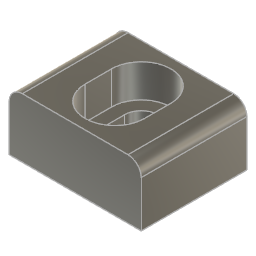
ZAxis Cap (Autodesk Fusion 360 design; units mm, degrees)
Autodesk Fusion 360 part; units mm, degrees
sketch "Sketch1" plane through (0, 0, 0) normal (0, 0, 1) x (1, 0, 0)
  line L0 (0, 0) -> (20, 0)
  line L1 (20, 0) -> (20, -16)
  line L2 (20, -16) -> (0, -16)
  line L3 (0, -16) -> (0, 0)
  line L4 (20, -8) -> (0, -8) construction
  line L5 (10, 0) -> (10, -16) construction
  line L6 (7.5, -6) -> (7.5, -10)
  arc A0 (7.5, -10) -> (12.5, -10) centre (10, -10) ccw
  line L7 (12.5, -10) -> (12.5, -6)
  arc A1 (12.5, -6) -> (7.5, -6) centre (10, -6) ccw
  line L8 (10, -6) -> (10, -10) construction
  line L9 (5.5, -6) -> (5.5, -10)
  arc A2 (5.5, -10) -> (14.5, -10) centre (10, -10) ccw
  line L10 (14.5, -10) -> (14.5, -6)
  arc A3 (14.5, -6) -> (5.5, -6) centre (10, -6) ccw
  line L11 (10, -6) -> (10, -10) construction
  dimension "d1" = 20
  dimension "d2" = 16
  dimension "d11" = 5
  dimension "d12" = 2
  dimension "d13" = 2
  dimension "d14" = 9
  constraint horizontal L0
  constraint vertical L1
  constraint horizontal L2
  constraint vertical L3
  constraint coincident L0.start L3.end
  constraint midpoint L1 L4.start
  constraint midpoint L3 L4.end
  constraint midpoint L0 L5.start
  constraint midpoint L2 L5.end
  constraint tangent L6 A0
  constraint tangent A0 L7
  constraint parallel L6 L7
  constraint tangent L7 A1
  constraint tangent L6 A1
  constraint perpendicular L4 L8
  constraint coincident L5 A1.centre
  constraint tangent L9 A2
  constraint tangent A2 L10
  constraint parallel L9 L10
  constraint tangent L10 A3
  constraint tangent L9 A3
  constraint coincident A0.centre L8.end
  constraint perpendicular L4 L11
  constraint coincident A1.centre L8.start
  measures "d1" distance of L0.start L0.end
  measures "d2" distance of L0.start L2.end
  measures "d11" diameter of A0
  measures "d12" distance of L4 A0.centre
  measures "d13" distance of L4 A1.centre
  measures "d14" diameter of A2
extrude "Extrude1" add sketch "Sketch1" along normal blind 4 contours L0 L1 L2 L3 | L9 A2 L10 A3
extrude "Extrude2" add sketch "Sketch1" along normal blind 5 from surface at 4 contours L0 L1 L2 L3
fillet "Fillet1" radius 2 2 edges at (20, -8, 9) (0, -8, 9)
